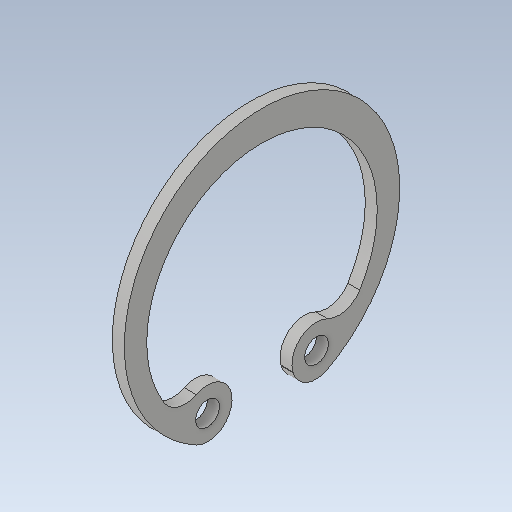
# Autodesk Inventor part: RRING-C-INT-S-22
Saved by Autodesk Inventor 2020.2 (Build 242310000, 310)
## iProperties
Created: 2022-11-04
Part Number: RRING-C-INT-S-22
Material: Generic
Catalog Web Link: www.cadenas.de
Description: RRING_C_INT-Retaining Rings - C  (Internal)
Vendor: MISUMI
Document SubType Name: Modeling
Designer: psAdmin
Manufacturer: MISUMI
Mass: 0.128626 g
Surface Area: 3.94561 cm^2
Volume: 0.128626 cm^3
Density: 1 g/cm^3
Appearance: PSOLRGB-175-175-175
Category: PARTsolutions
Company: MISUMI
PSOL_IDENT_0: {$CADENAS_DATA/23d-libs/misumi/metric/accessories/rring_c_int.prj},181 {VTYP=3D},{NB=RRING-C-INT-S-2
PSOL_IDENT_1: 2},{LINA=RRING-C-INT-S-22},{NN=RRING_C_INT},{DATE=30.06.2021 13:30:10},{GEOMDATE=05.03.2015 00:00:00
PSOL_IDENT_2: },{VERSION=},{LINEID=120},{WBVAR=MAT},{WBNUMERIC=}  {NB=RRING-C-INT-S-22},{LINA=RRING-C-INT-S-22},{K
PSOL_IDENT_3: T=DUMMY},{PN=RRING-C-INT-S-22},{TYPE=RRING-C-INT},{MAT=-S},{HARD=36~44HRC},{NO=22},{DD3=23.5},{DD3TO
PSOL_IDENT_4: L=+0.2/-0.2},{TT=1.00},{TTTOL=+0.05/-0.05},{BB=2.5},{AA=4.1},{DD0=2.0},{DD4=13},{DD1=22},{DD2=23.0},
PSOL_IDENT_5: {DD2TOL=+0.21/0},{MM=1.15},{MMTOL=+0.14/0},{NN=1.5},{A2=9.10}
NB: RRING-C-INT-S-22
NN: 1.5
NT: Retaining Rings - C  (Internal)
NBSYN: $PN.
LINA: RRING-C-INT-S-22
CATALOG: Misumi
PN: RRING-C-INT-S-22
MAT: 304 Stainless Steel-CSP
HARD: 36~44HRC
NO: 22
DD3: 23.5
DD3TOL: +0.2/-0.2
TT: 1
TTTOL: +0.05/-0.05
BB: 2.5
AA: 4.1
DD0: 2
DD4: 13
DD1: 22
DD2: 23
DD2TOL: +0.21/0
MM: 1.15
MMTOL: +0.14/0
SUPPLIER: MISUMI
ARTICLENO: RRING-C-INT-S-22
BOMINFO: RRING-C-INT-S-22
CREATOR: CADENAS GmbH
Title: RRING-C-INT-S-22
Author: Cadenas PARTsolutions
Comments: Retaining Rings - C  (Internal)
Autodesk Inventor part; units mm, degrees
sketch "Sketch_3" plane through (0, 0, 0) normal (1, 0, 0) x (0, 1, 0)
  arc A0 (-10.1153, -5.4708) -> (-10.1153, 5.4708) centre (0, 0) ccw
  arc A1 (-10.1153, 5.4708) -> (-8.9159, 2.5993) centre (-8.3561, 4.5194) ccw
  line L0 (-8.9159, 2.5993) -> (-8.8563, 2.5819)
  arc A2 (-8.8563, 2.5819) -> (-6.4596, 5.4878) centre (-8.2825, 4.55) ccw
  arc A3 (-5.7223, 8.1644) -> (-6.4596, 5.4878) centre (-4.6366, 6.4255) ccw
  arc A4 (-5.7223, -8.1644) -> (-5.7223, 8.1644) centre (-0.625, 0) ccw
  arc A5 (-6.4596, -5.4878) -> (-5.7223, -8.1644) centre (-4.6366, -6.4255) ccw
  arc A6 (-6.4596, -5.4878) -> (-8.8563, -2.5819) centre (-8.2825, -4.55) ccw
  line L1 (-8.8563, -2.5819) -> (-8.9159, -2.5993)
  arc A7 (-8.9159, -2.5993) -> (-10.1153, -5.4708) centre (-8.3561, -4.5194) ccw
  circle A8 centre (-8.2825, -4.55) radius 1
  circle A9 centre (-8.2825, 4.55) radius 1
  constraints: 16 point on circle, 10 centre point, 4 end point
extrude "Extrusion1" add sketch "Sketch_3" along normal mid plane 1
ref_plane "rr_XY" through (-0.5, 0, 0) normal (1, 0, 0) x (0, 0, -1)
ref_plane "rr_YZ" through (-0.5, 0, 0) normal (0, 0, -1) x (0, 1, 0)
ref_plane "rr_ZX" through (-0.5, 0, 0) normal (0, 1, 0) x (1, 0, 0)
body "Solid1"
